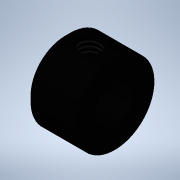
# Autodesk Inventor part: 623890046_1
Saved by Autodesk Inventor 2021 (Build 250183000, 183)
## iProperties
Created: 2026-04-17
Part Number: 623890046_1
Material: Generic
Catalog Web Link: www.3dfindit.com
Description: rohteil_din705_a-Raw part, Adjusting Rings (Shaft Collars with Set Screw)  DIN 705 A
Vendor: MAEDLER
Document SubType Name: Modeling
Designer: psAdmin
Manufacturer: MAEDLER
Mass: 0.178848 g
Surface Area: 2.6103 cm^2
Volume: 0.178848 cm^3
Density: 1 g/cm^3
Appearance: PSOLRGB-44-44-44
Category: PARTsolutions
Company: MAEDLER
Title: 623890046
Author: Cadenas PARTsolutions
Comments: Raw part, Adjusting Rings (Shaft Collars with Set Screw)  DIN 705 A
PSOL_IDENT_0: {$CADENAS_DATA/23d-libs/maedler/antriebselemente/klemmringe_stellringe/stellringe/din705a/din_705a_i
PSOL_IDENT_1: s_4027/rohteil_din705_a.prj},172 {VTYP=3D},{NB=623890046_1},{LINA=623890046},{NN=rohteil_din705_a},{
PSOL_IDENT_2: DATE=01.12.2025 10:57:12},{GEOMDATE=04.08.2024 15:45:00},{VERSION=},{LINEID=2580},{WBVAR=},{WBNUMERI
PSOL_IDENT_3: C=}  {NB=623890046_1},{LINA=623890046},{KT=DUMMY},{ARTNR=623890046},{WEBSHOP=Produktdetails / Katalo
PSOL_IDENT_4: gseite / Montageanleitung},{MATK=Stahl brüniert},{MAT=Stahl brüniert, Gewindestift mit Festigkeit 45
PSOL_IDENT_5: H oder 12.9, schwarz},{AUSF=mit 1x Gewindestift mit Innensechskant DIN EN ISO 4027},{D1=4},{D2=8},{B=
PSOL_IDENT_6: 5},{SCHR=M2,5 x 3},{GEW=0.152},{D3=2.010},{SCHRAUBE=2.5},{DD1=0.00},{N=0.0},{T=0.0},{DDD1=0.7},{SW=1
PSOL_IDENT_7: .3},{T1=1.2},{SCHRL=3},{SCHRUEB=1.0},{TYP=2},{CTN=73182900},{DIST=0.52},{CNSDWTEMPLATE=_dw/ansicht_f
PSOL_IDENT_8: ront_left.dw}
NB: 623890046_1
NN: rohteil_din705_a
NT: Raw part, Adjusting Rings (Shaft Collars with Set Screw)  DIN 705 A
NBSYN: $ARTNR._1
LINA: 623890046
CATALOG: MÄDLER
ARTNR: 623890046
WEBSHOP: Product details / Catalogue page / Assembly instructions
MATK: Steel, black oxide finish
MAT: Steel, black oxide finish, Set screw with strength 45H or 12.9, black
AUSF: with 1x Set screw with hexagon socket DIN EN ISO 4027
D1: 4
D2: 8
B: 5
SCHR: M2,5 x 3
GEW: 0.152
D3: 2.01
SCHRAUBE: 2.5
DD1: 0
N: 0
T: 0
DDD1: 0.7
SW: 1.3
T1: 1.2
SCHRL: 3
SCHRUEB: 1
TYP: 2
CTN: 73182900
SUPPLIER: MAEDLER
ARTICLENO: 623890046_1
BOMINFO: 623890046
CREATOR: CADENAS GmbH
Autodesk Inventor part; units mm, degrees
sketch "Skizze_1" plane through (0, 0, 0) normal (0, 0, 1) x (1, 0, 0)
  line L0 (2.5, 0) -> (-2.5, 0)
  line L1 (-2.5, 3.5) -> (-2.5, 2.0707)
  line L2 (-2.5, 2.0707) -> (-2.4293, 2)
  line L3 (-2.4293, 2) -> (2.4293, 2)
  line L4 (2.4293, 2) -> (2.5, 2.0707)
  line L5 (2.5, 2.0707) -> (2.5, 4)
  line L6 (2.5, 4) -> (-2, 4)
  line L7 (-2, 4) -> (-2.5, 3.5)
  constraints: 16 end point
revolve "Revolution1" add sketch "Skizze_1" angle 360 about axis through (2.5, 0, 0) along (1, 0, 0)
sketch "Skizze_2" plane through (0, 0, 0) normal (0, 0, 1) x (1, 0, 0)
  line L0 (0, 1.25) -> (0, 4)
  line L1 (0, 4) -> (1.25, 4)
  line L2 (1.25, 4) -> (1.0065, 3.7565)
  line L3 (1.0065, 3.7565) -> (1.0065, 1.4935)
  line L4 (1.0065, 1.4935) -> (1.25, 1.25)
  line L5 (1.25, 1.25) -> (0, 1.25)
  line L6 (0, 1.25) -> (0, 4)
  constraints: 14 end point
revolve "Revolution2" cut sketch "Skizze_2" angle 360 about axis through (0, 1.25, 0) along (0, -1, 0)
thread "Thread1" size "M2.5x0.45" class "6H" standard "ISO Metric profile" length 2.263
ref_plane "gst_nr_1_XY" through (0, 4, 0) normal (0, 1, 0) x (1, 0, 0)
ref_plane "gst_nr_1_YZ" through (0, 4, 0) normal (1, 0, 0) x (0, 0, -1)
ref_plane "gst_nr_1_ZX" through (0, 4, 0) normal (0, 0, -1) x (0, 1, 0)
body "Solid1"
